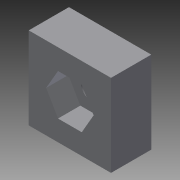
# Autodesk Inventor part: BoltTrace
Saved by Autodesk Inventor 2014 (Build 180170000, 170)
## iProperties
Created: 2013-09-18
Part Number: BoltTrace
Material: Generic
Document SubType Name: Modeling
Designer: Medrimonia
Density: 1 g/cm^3
Appearance: Default
Author: Medrimonia
Autodesk Inventor part; units mm, degrees
ref_plane "YZ Plane" through (0, 0, 0) normal (1, 0, 0) x (0, 1, 0)
ref_plane "XZ Plane" through (0, 0, 0) normal (0, 1, 0) x (-1, 0, 0)
ref_plane "XY Plane" through (0, 0, 0) normal (0, 0, 1) x (1, 0, 0)
sketch "Sketch1" plane through (0, 0, 0) normal (0, 1, 0) x (-1, 0, 0)
  line L0 (-4.6, 4.6) -> (4.6, 4.6)
  line L1 (4.6, 4.6) -> (4.6, -4.6)
  line L2 (4.6, -4.6) -> (-4.6, -4.6)
  line L3 (-4.6, -4.6) -> (-4.6, 4.6)
  point P0 (0, 0)
  dimension "d0" = 9.2
  dimension "d1" = 9.2
  dimension "d2" = 4.6
  dimension "d3" = 4.6
  constraints: 8 end point, 2 parallel, 1 horizontal, 1 perpendicular
  measures "d0" distance of L0.end L1.end
  measures "d1" distance of L0.start L0.end
  measures "d2" distance from line of L1 point (0, 0)
  measures "d3" distance from line of L0 point (0, 0)
extrude "Extrusion1" add sketch "Sketch1" along normal blind 4.5
sketch "Sketch3" plane through (0, 0, 0) normal (0, -1, 0) x (1, 0, 0)
  line L0 (-4.6, -4.6) -> (4.6, -4.6) projected
  line L1 (-4.6, 4.6) -> (4.6, -4.6) construction
  line L2 (4.6, 4.6) -> (-4.6, -4.6) construction
  line L3 (1.3279, 2.3) -> (2.6558, 0)
  line L4 (2.6558, 0) -> (1.3279, -2.3)
  line L5 (1.3279, -2.3) -> (-1.3279, -2.3)
  line L6 (-1.3279, -2.3) -> (-2.6558, 0)
  line L7 (-2.6558, 0) -> (-1.3279, 2.3)
  line L8 (-1.3279, 2.3) -> (1.3279, 2.3)
  point P0 (0, 0)
  point P1 (0, 0)
  dimension "d7" = 4.6
  constraints: 16 end point, 1 coincident, 1 parallel, 1 perpendicular, 13 other
  measures "d7" distance between parallel lines of L5 L8
extrude "Extrusion2" cut sketch "Sketch3" against normal blind 2.5
sketch "Sketch4" plane through (0, 4.5, 0) normal (0, 1, 0) x (1, 0, 0)
  circle A0 centre (0, 0) radius 1.3
  dimension "d10" = 2.6
  constraints: 1 centre point, 1 coincident
  measures "d10" diameter of A0
extrude "Extrusion3" cut sketch "Sketch4" against normal blind 2
equation "\"d0\" = 2 * BoltTrace"
equation "\"d1\" = d0"
equation "\"d2\" = 0.5 * d1"
equation "\"d3\" = 0.5 * d0"
equation "\"d4\" = ClassicThickness"
equation "\"d7\" = BoltTrace"
equation "\"d8\" = BoltThickness"
equation "\"d10\" = ServoScrewDiameterRequired"
equation "\"d11\" = MinimalThickness"
equation "\"BoltTrace\" = 4.6"
equation "\"ClassicThickness\" = 4.5"
equation "\"BoltThickness\" = 2.5"
equation "\"ServoScrewDiameterRequired\" = 2.6"
equation "\"MinimalThickness\" = 2"
body "Solid1"
